Autodesk Fusion 360 part; units mm, degrees
(part 2 of 2)
  dimension "d128" = 3
  constraint coincident A32.centre A41.centre
  constraint coincident A25.centre A40.centre
  constraint coincident A38.centre A43.centre
  constraint coincident A34.centre A42.centre
  measures "d125" diameter of A21
  measures "d126" diameter of A23
  measures "d127" diameter of A24
  measures "d128" diameter of A22
extrude "Extrude11" cut sketch "Sketch4" against normal blind 8 contours A21 | A22 | A23 | A24
extrude "Extrude12" cut sketch "Sketch4" against normal blind 6.5 contours A25 | A32 | A34 | A38 | A40 | A41 | A42 | A43
sketch "Sketch5" plane through (0, 0, 3) normal (0, 0, 1) x (-1, 0, 0)
  circle A0 centre (47, -22) radius 1.5
  circle A1 centre (19.8064, 49.2459) radius 1.5
  circle A2 centre (-21.042, -45.9567) radius 1.5
  circle A3 centre (-47.207, 20.5835) radius 1.5
  circle A4 centre (14, -47) radius 1.5
  circle A5 centre (-47, -14) radius 1.5
  circle A6 centre (47, 14) radius 1.5
  circle A7 centre (-14, 47) radius 1.5
  arc A8 (55, 15) -> (15, 55) centre (15, 15) ccw
  line L0 (15, 55) -> (-15, 55)
  arc A9 (-15, 55) -> (-55, 15) centre (-15, 15) ccw
  line L1 (-55, 15) -> (-55, -15)
  arc A10 (-55, -15) -> (-15, -55) centre (-15, -15) ccw
  line L2 (-15, -55) -> (15, -55)
  arc A11 (15, -55) -> (55, -15) centre (15, -15) ccw
  line L3 (55, -15) -> (55, 15)
  line L4 (41.4394, -9.8393) -> (37.3179, -15.2919)
  spline S0 degree 3 poles (37.3179, -15.2919) (37.6885, -19.157) (38.1371, -22.7222) (37.3203, -26.0559) (37.037, -26.7219) (36.2871, -27.772) (35.8641, -28.165) (34.6133, -28.9678) (33.7328, -29.2635) (32.7908, -29.4916) knots 0 0 0 0 1.164828 1.164828 1.516946 1.516946 1.81941 1.81941 2.270031 2.270031 2.270031 2.270031
  line L5 (32.7908, -29.4916) -> (31.7989, -35.8027)
  line L6 (31.7989, -35.8027) -> (31.0974, -40.2607)
  line L7 (31.0974, -40.2607) -> (33.5883, -40.8482)
  line L8 (33.5883, -40.8482) -> (32.8996, -43.7681)
  line L9 (32.8996, -43.7681) -> (30.6297, -43.2327)
  line L10 (30.6297, -43.2327) -> (29.9635, -47.4663)
  arc A12 (24.1405, -46.0928) -> (29.9635, -47.4663) centre (27, -47) ccw
  line L11 (24.1405, -46.0928) -> (25.4365, -42.0077)
  line L12 (25.4365, -42.0077) -> (23.1667, -41.4723)
  line L13 (23.1667, -41.4723) -> (23.8554, -38.5524)
  line L14 (23.8554, -38.5524) -> (26.3463, -39.14)
  line L15 (26.3463, -39.14) -> (27.7111, -34.8384)
  line L16 (27.7111, -34.8384) -> (28.7703, -30.3481)
  spline S1 degree 3 poles (28.7703, -30.3481) (27.6148, -30.6643) (26.6336, -31.0889) (24.9398, -32.4102) (24.298, -33.1659) (22.092, -36.2546) (20.5653, -39.283) (15.8311, -43.4069) (14.0247, -44.4113) (11.1819, -45.3972) (9.9898, -45.607) (8.1404, -45.5368) (7.3989, -45.3892) (6.1398, -44.8148) (5.64, -44.4531) (4.7208, -43.4815) (4.3496, -42.8831) (3.4629, -41.0501) (3.1013, -39.695) (2.3137, -37.6472) (1.9455, -36.8825) (1.0366, -35.7978) (0.5937, -35.4393) (-0.469, -34.89) (-1.0783, -34.7097) (-3.396, -34.3697) (-5.3987, -34.5812) (-7.6106, -34.9389) knots 0 0 0 0 0.359374 0.359374 0.670478 0.670478 1.446599 1.446599 1.895417 1.895417 2.224922 2.224922 2.450473 2.450473 2.63972 2.63972 2.850158 2.850158 3.247941 3.247941 3.519478 3.519478 3.715617 3.715617 3.915643 3.915643 4.385468 4.385468 4.385468 4.385468
  line L17 (-7.6106, -34.9389) -> (-5.7671, -36.87)
  line L18 (-5.7671, -36.87) -> (-2.4134, -39.8897)
  line L19 (-2.4134, -39.8897) -> (-0.5622, -38.1225)
  line L20 (-0.5622, -38.1225) -> (1.5093, -40.2925)
  line L21 (1.5093, -40.2925) -> (-0.1776, -41.9029)
  line L22 (-0.1776, -41.9029) -> (3.0074, -44.7706)
  arc A13 (-1.3202, -48.9018) -> (3.0074, -44.7706) centre (1, -47) ccw
  line L23 (-1.3202, -48.9018) -> (-4.037, -45.5872)
  line L24 (-4.037, -45.5872) -> (-5.7239, -47.1976)
  line L25 (-5.7239, -47.1976) -> (-7.7954, -45.0276)
  line L26 (-7.7954, -45.0276) -> (-5.9442, -43.2604)
  line L27 (-5.9442, -43.2604) -> (-12.1168, -35.7299)
  spline S2 degree 3 poles (-12.1168, -35.7299) (-14.7803, -36.1844) (-17.4077, -36.5262) (-20.6177, -36.1408) (-21.5954, -35.8949) (-23.1516, -35.0659) (-23.7332, -34.592) (-24.6878, -33.4235) (-25.0394, -32.7732) (-25.5995, -31.3254) (-25.7916, -30.5154) (-25.9192, -29.7135) knots 0 0 0 0 0.810588 0.810588 1.168868 1.168868 1.446193 1.446193 1.71283 1.71283 2.006296 2.006296 2.006296 2.006296
  line L28 (-25.9192, -29.7135) -> (-35.1529, -29.8382)
  line L29 (-35.1529, -29.8382) -> (-39.6653, -29.8999)
  line L30 (-39.6653, -29.8999) -> (-39.8236, -32.4543)
  line L31 (-39.8236, -32.4543) -> (-42.8179, -32.2688)
  line L32 (-42.8179, -32.2688) -> (-42.6736, -29.9411)
  line L33 (-42.6736, -29.9411) -> (-46.959, -29.9997)
  arc A14 (-46.5889, -24.0283) -> (-46.959, -29.9997) centre (-47, -27) ccw
  line L34 (-46.5889, -24.0283) -> (-42.3436, -24.6156)
  line L35 (-42.3436, -24.6156) -> (-42.1994, -22.2879)
  line L36 (-42.1994, -22.2879) -> (-39.2051, -22.4735)
  line L37 (-39.2051, -22.4735) -> (-39.3634, -25.0279)
  line L38 (-39.3634, -25.0279) -> (-34.8931, -25.6463)
  line L39 (-34.8931, -25.6463) -> (-26.1751, -26.1865)
  spline S3 degree 3 poles (-26.1751, -26.1865) (-26.2136, -21.5897) (-25.4228, -16.5889) (-26.5447, -7.6817) (-27.7362, -4.5994) (-31.4465, 2.9635) (-33.9112, 7.1935) (-35.421, 11.5615) knots 0 0 0 0 1.379101 1.379101 2.416171 2.416171 3.558045 3.558045 3.558045 3.558045
  line L40 (-35.421, 11.5615) -> (-38.3057, 7.5335)
  line L41 (-38.3057, 7.5335) -> (-40.6488, 3.6765)
  line L42 (-40.6488, 3.6765) -> (-38.5681, 2.1864)
  line L43 (-38.5681, 2.1864) -> (-40.3148, -0.2527)
  line L44 (-40.3148, -0.2527) -> (-42.2109, 1.1052)
  line L45 (-42.2109, 1.1052) -> (-44.436, -2.5576)
  arc A15 (-49.3002, 0.9259) -> (-44.436, -2.5576) centre (-47, -1) ccw
  line L46 (-49.3002, 0.9259) -> (-46.5489, 4.2119)
  line L47 (-46.5489, 4.2119) -> (-48.445, 5.5698)
  line L48 (-48.445, 5.5698) -> (-46.6982, 8.0088)
  line L49 (-46.6982, 8.0088) -> (-44.6175, 6.5187)
  line L50 (-44.6175, 6.5187) -> (-41.7204, 9.9789)
  line L51 (-41.7204, 9.9789) -> (-36.6853, 17.0096)
  spline S4 degree 3 poles (-36.6853, 17.0096) (-36.8676, 18.8531) (-36.7596, 20.6853) (-35.8249, 23.83) (-35.1927, 25.0859) (-33.4931, 27.4447) (-32.4383, 28.4998) (-31.2814, 29.4234) knots 0 0 0 0 0.555731 0.555731 0.983651 0.983651 1.42815 1.42815 1.42815 1.42815
  line L52 (-31.2814, 29.4234) -> (-30.8456, 35.4405)
  line L53 (-30.8456, 35.4405) -> (-30.5194, 39.9416)
  line L54 (-30.5194, 39.9416) -> (-33.0508, 40.3188)
  line L55 (-33.0508, 40.3188) -> (-32.6086, 43.286)
  line L56 (-32.6086, 43.286) -> (-30.3019, 42.9423)
  line L57 (-30.3019, 42.9423) -> (-29.9922, 47.2169)
  arc A16 (-24.0746, 46.3351) -> (-29.9922, 47.2169) centre (-27, 47) ccw
  line L58 (-24.0746, 46.3351) -> (-25.0245, 42.156)
  line L59 (-25.0245, 42.156) -> (-22.7178, 41.8122)
  line L60 (-22.7178, 41.8122) -> (-23.16, 38.845)
  line L61 (-23.16, 38.845) -> (-25.6913, 39.2222)
  line L62 (-25.6913, 39.2222) -> (-26.6915, 34.8215)
  line L63 (-26.6915, 34.8215) -> (-27.102, 32.0663)
  spline S5 degree 3 poles (-27.102, 32.0663) (-23.8561, 33.7038) (-20.1727, 34.7945) (-13.9908, 35.6095) (-11.9033, 35.3478) (-8.6393, 34.4929) (-7.241, 33.737) (-4.6779, 32.215) (-3.539, 31.4712) (-1.7666, 30.8258) (-1.1355, 30.6903) (0.1203, 30.7222) (0.6844, 30.8607) (1.9595, 31.399) (2.6674, 31.8714) (4.3852, 33.2548) (5.4117, 34.2687) (6.5195, 35.3415) knots 0 0 0 0 1.090679 1.090679 2.116632 2.116632 3.315493 3.315493 4.459674 4.459674 5.071625 5.071625 5.626071 5.626071 6.359803 6.359803 7.369828 7.369828 7.369828 7.369828
  line L64 (6.5195, 35.3415) -> (5.3836, 36.6241)
  line L65 (5.3836, 36.6241) -> (2.1451, 39.7671)
  line L66 (2.1451, 39.7671) -> (0.2292, 38.0703)
  line L67 (0.2292, 38.0703) -> (-1.7598, 40.3162)
  line L68 (-1.7598, 40.3162) -> (-0.0138, 41.8624)
  line L69 (-0.0138, 41.8624) -> (-3.0893, 44.8472)
  arc A17 (1.3897, 48.8137) -> (-3.0893, 44.8472) centre (-1, 47) ccw
  line L70 (1.3897, 48.8137) -> (3.9807, 45.3999)
  line L71 (3.9807, 45.3999) -> (5.7266, 46.946)
  line L72 (5.7266, 46.946) -> (7.7155, 44.7001)
  line L73 (7.7155, 44.7001) -> (5.7996, 43.0034)
  line L74 (5.7996, 43.0034) -> (8.5279, 39.4086)
  line L75 (8.5279, 39.4086) -> (9.6251, 38.1696)
  spline S6 degree 3 poles (9.6251, 38.1696) (11.2124, 39.4725) (12.9202, 40.5975) (16.4323, 41.9003) (18.0613, 42.1653) (21.4266, 42.0265) (23.0731, 41.6295) (26.5653, 40.2029) (28.3145, 39.0547) (30.2985, 37.2379) (30.8783, 36.6163) (31.7822, 35.4004) (32.1434, 34.8061) (32.416, 34.173) knots 0 0 0 0 0.616058 0.616058 1.127035 1.127035 1.633478 1.633478 2.269407 2.269407 2.553154 2.553154 2.787926 2.787926 2.787926 2.787926
  line L76 (32.416, 34.173) -> (36.3135, 32.8488)
  line L77 (36.3135, 32.8488) -> (40.6839, 31.7237)
  line L78 (40.6839, 31.7237) -> (41.5072, 34.147)
  line L79 (41.5072, 34.147) -> (44.3477, 33.1819)
  line L80 (44.3477, 33.1819) -> (43.5975, 30.9737)
  line L81 (43.5975, 30.9737) -> (47.7479, 29.9053)
  arc A18 (45.8232, 24.2404) -> (47.7479, 29.9053) centre (47, 27) ccw
  line L82 (45.8232, 24.2404) -> (41.881, 25.9216)
  line L83 (41.881, 25.9216) -> (41.1307, 23.7134)
  line L84 (41.1307, 23.7134) -> (38.2902, 24.6785)
  line L85 (38.2902, 24.6785) -> (39.1135, 27.1018)
  line L86 (39.1135, 27.1018) -> (34.9623, 28.872)
  line L87 (34.9623, 28.872) -> (33.0026, 29.5379)
  spline S7 degree 3 poles (33.0026, 29.5379) (32.9902, 28.5579) (33.003, 27.1751) (33.5348, 25.6326) (33.7207, 25.3268) (34.1024, 24.8702) (34.3236, 24.7044) (34.8418, 24.4372) (35.1527, 24.347) (36.4443, 24.0711) (37.7665, 23.9707) (40.2586, 22.8614) (41.1591, 22.2488) (42.5804, 20.7638) (43.1055, 19.9446) (43.8206, 18.0888) (43.9818, 17.0988) (44.0027, 14.699) (43.7263, 13.2998) (42.5231, 9.2938) (41.1447, 6.638) (39.093, 2.0196) (38.3333, 0.1029) (37.2326, -4.3021) (36.9907, -6.4921) (36.9644, -8.7943) knots 0 0 0 0 0.294006 0.294006 0.417435 0.417435 0.550082 0.550082 0.704478 0.704478 1.129194 1.129194 1.408869 1.408869 1.66214 1.66214 1.922723 1.922723 2.2812 2.2812 3.001747 3.001747 3.492602 3.492602 4.002499 4.002499 4.002499 4.002499
  line L88 (36.9644, -8.7943) -> (38.0888, -7.3067)
  line L89 (38.0888, -7.3067) -> (40.5305, -3.5114)
  line L90 (40.5305, -3.5114) -> (38.4888, -1.9682)
  line L91 (38.4888, -1.9682) -> (40.2978, 0.4251)
  line L92 (40.2978, 0.4251) -> (42.1583, -0.9812)
  line L93 (42.1583, -0.9812) -> (44.477, 2.6231)
  arc A19 (49.2498, -0.9845) -> (44.477, 2.6231) centre (47, 1) ccw
  line L94 (49.2498, -0.9845) -> (46.4148, -4.1986)
  line L95 (46.4148, -4.1986) -> (48.2753, -5.6048)
  line L96 (48.2753, -5.6048) -> (46.4663, -7.9981)
  line L97 (46.4663, -7.9981) -> (44.4246, -6.4548)
  line L98 (44.4246, -6.4548) -> (41.4394, -9.8393)
  circle A20 centre (37.75, -38.15) radius 2.75
  circle A21 centre (38.15, 37.75) radius 2.75
  circle A22 centre (-38.15, -37.75) radius 2.75
  circle A23 centre (-37.75, 38.15) radius 2.75
  circle A24 centre (19.8064, 49.2459) radius 4
  line L99 (23.8064, 49.2459) -> (23.8064, 54.0186)
  line L100 (15.8064, 49.2459) -> (15.8064, 54.9919)
  dimension "d133" = 8
  constraint concentric A1 A24
  constraint coincident A24 L99.start
  constraint coincident A8 L99.end
  constraint tangent A24 L99
  constraint vertical L99
  constraint coincident A24 L100.start
  constraint coincident A8 L100.end
  constraint tangent A24 L100
  constraint vertical L100
  measures "d133" diameter of A24
sketch "LaserMidPlateShellBearing" plane through (0, 0, 3) normal (0, 0, 1) x (-1, 0, 0)
  circle A0 centre (47, -22) radius 1.5
  circle A1 centre (19.8064, 49.2459) radius 1.5
  circle A2 centre (-21.042, -45.9567) radius 1.5
  circle A3 centre (-47.207, 20.5835) radius 1.5
  circle A4 centre (14, -47) radius 1.5
  circle A5 centre (-47, -14) radius 1.5
  circle A6 centre (47, 14) radius 1.5
  circle A7 centre (-14, 47) radius 1.5
  arc A8 (55, 15) -> (15, 55) centre (15, 15) ccw
  line L0 (15, 55) -> (-15, 55)
  arc A9 (-15, 55) -> (-55, 15) centre (-15, 15) ccw
  line L1 (-55, 15) -> (-55, -15)
  arc A10 (-55, -15) -> (-15, -55) centre (-15, -15) ccw
  line L2 (-15, -55) -> (15, -55)
  arc A11 (15, -55) -> (55, -15) centre (15, -15) ccw
  line L3 (55, -15) -> (55, 15)
  line L4 (41.4394, -9.8393) -> (37.3179, -15.2919)
  spline S0 degree 3 poles (37.3179, -15.2919) (37.6885, -19.157) (38.1371, -22.7222) (37.3203, -26.0559) (37.037, -26.7219) (36.2871, -27.772) (35.8641, -28.165) (34.6133, -28.9678) (33.7328, -29.2635) (32.7908, -29.4916) knots 0 0 0 0 1.164828 1.164828 1.516946 1.516946 1.81941 1.81941 2.270031 2.270031 2.270031 2.270031
  line L5 (32.7908, -29.4916) -> (31.7989, -35.8027)
  line L6 (31.7989, -35.8027) -> (31.0974, -40.2607)
  line L7 (31.0974, -40.2607) -> (33.5883, -40.8482)
  line L8 (33.5883, -40.8482) -> (32.8996, -43.7681)
  line L9 (32.8996, -43.7681) -> (30.6297, -43.2327)
  line L10 (30.6297, -43.2327) -> (29.9635, -47.4663)
  arc A12 (24.1405, -46.0928) -> (29.9635, -47.4663) centre (27, -47) ccw
  line L11 (24.1405, -46.0928) -> (25.4365, -42.0077)
  line L12 (25.4365, -42.0077) -> (23.1667, -41.4723)
  line L13 (23.1667, -41.4723) -> (23.8554, -38.5524)
  line L14 (23.8554, -38.5524) -> (26.3463, -39.14)
  line L15 (26.3463, -39.14) -> (27.7111, -34.8384)
  line L16 (27.7111, -34.8384) -> (28.7703, -30.3481)
  spline S1 degree 3 poles (28.7703, -30.3481) (27.6148, -30.6643) (26.6336, -31.0889) (24.9398, -32.4102) (24.298, -33.1659) (22.092, -36.2546) (20.5653, -39.283) (15.8311, -43.4069) (14.0247, -44.4113) (11.1819, -45.3972) (9.9898, -45.607) (8.1404, -45.5368) (7.3989, -45.3892) (6.1398, -44.8148) (5.64, -44.4531) (4.7208, -43.4815) (4.3496, -42.8831) (3.4629, -41.0501) (3.1013, -39.695) (2.3137, -37.6472) (1.9455, -36.8825) (1.0366, -35.7978) (0.5937, -35.4393) (-0.469, -34.89) (-1.0783, -34.7097) (-3.396, -34.3697) (-5.3987, -34.5812) (-7.6106, -34.9389) knots 0 0 0 0 0.359374 0.359374 0.670478 0.670478 1.446599 1.446599 1.895417 1.895417 2.224922 2.224922 2.450473 2.450473 2.63972 2.63972 2.850158 2.850158 3.247941 3.247941 3.519478 3.519478 3.715617 3.715617 3.915643 3.915643 4.385468 4.385468 4.385468 4.385468
  line L17 (-7.6106, -34.9389) -> (-5.7671, -36.87)
  line L18 (-5.7671, -36.87) -> (-2.4134, -39.8897)
  line L19 (-2.4134, -39.8897) -> (-0.5622, -38.1225)
  line L20 (-0.5622, -38.1225) -> (1.5093, -40.2925)
  line L21 (1.5093, -40.2925) -> (-0.1776, -41.9029)
  line L22 (-0.1776, -41.9029) -> (3.0074, -44.7706)
  arc A13 (-1.3202, -48.9018) -> (3.0074, -44.7706) centre (1, -47) ccw
  line L23 (-1.3202, -48.9018) -> (-4.037, -45.5872)
  line L24 (-4.037, -45.5872) -> (-5.7239, -47.1976)
  line L25 (-5.7239, -47.1976) -> (-7.7954, -45.0276)
  line L26 (-7.7954, -45.0276) -> (-5.9442, -43.2604)
  line L27 (-5.9442, -43.2604) -> (-12.1168, -35.7299)
  spline S2 degree 3 poles (-12.1168, -35.7299) (-14.7803, -36.1844) (-17.4077, -36.5262) (-20.6177, -36.1408) (-21.5954, -35.8949) (-23.1516, -35.0659) (-23.7332, -34.592) (-24.6878, -33.4235) (-25.0394, -32.7732) (-25.5995, -31.3254) (-25.7916, -30.5154) (-25.9192, -29.7135) knots 0 0 0 0 0.810588 0.810588 1.168868 1.168868 1.446193 1.446193 1.71283 1.71283 2.006296 2.006296 2.006296 2.006296
  line L28 (-25.9192, -29.7135) -> (-35.1529, -29.8382)
  line L29 (-35.1529, -29.8382) -> (-39.6653, -29.8999)
  line L30 (-39.6653, -29.8999) -> (-39.8236, -32.4543)
  line L31 (-39.8236, -32.4543) -> (-42.8179, -32.2688)
  line L32 (-42.8179, -32.2688) -> (-42.6736, -29.9411)
  line L33 (-42.6736, -29.9411) -> (-46.959, -29.9997)
  arc A14 (-46.5889, -24.0283) -> (-46.959, -29.9997) centre (-47, -27) ccw
  line L34 (-46.5889, -24.0283) -> (-42.3436, -24.6156)
  line L35 (-42.3436, -24.6156) -> (-42.1994, -22.2879)
  line L36 (-42.1994, -22.2879) -> (-39.2051, -22.4735)
  line L37 (-39.2051, -22.4735) -> (-39.3634, -25.0279)
  line L38 (-39.3634, -25.0279) -> (-34.8931, -25.6463)
  line L39 (-34.8931, -25.6463) -> (-26.1751, -26.1865)
  spline S3 degree 3 poles (-26.1751, -26.1865) (-26.2136, -21.5897) (-25.4228, -16.5889) (-26.5447, -7.6817) (-27.7362, -4.5994) (-31.4465, 2.9635) (-33.9112, 7.1935) (-35.421, 11.5615) knots 0 0 0 0 1.379101 1.379101 2.416171 2.416171 3.558045 3.558045 3.558045 3.558045
  line L40 (-35.421, 11.5615) -> (-38.3057, 7.5335)
  line L41 (-38.3057, 7.5335) -> (-40.6488, 3.6765)
  line L42 (-40.6488, 3.6765) -> (-38.5681, 2.1864)
  line L43 (-38.5681, 2.1864) -> (-40.3148, -0.2527)
  line L44 (-40.3148, -0.2527) -> (-42.2109, 1.1052)
  line L45 (-42.2109, 1.1052) -> (-44.436, -2.5576)
  arc A15 (-49.3002, 0.9259) -> (-44.436, -2.5576) centre (-47, -1) ccw
  line L46 (-49.3002, 0.9259) -> (-46.5489, 4.2119)
  line L47 (-46.5489, 4.2119) -> (-48.445, 5.5698)
  line L48 (-48.445, 5.5698) -> (-46.6982, 8.0088)
  line L49 (-46.6982, 8.0088) -> (-44.6175, 6.5187)
  line L50 (-44.6175, 6.5187) -> (-41.7204, 9.9789)
  line L51 (-41.7204, 9.9789) -> (-36.6853, 17.0096)
  spline S4 degree 3 poles (-36.6853, 17.0096) (-36.8676, 18.8531) (-36.7596, 20.6853) (-35.8249, 23.83) (-35.1927, 25.0859) (-33.4931, 27.4447) (-32.4383, 28.4998) (-31.2814, 29.4234) knots 0 0 0 0 0.555731 0.555731 0.983651 0.983651 1.42815 1.42815 1.42815 1.42815
  line L52 (-31.2814, 29.4234) -> (-30.8456, 35.4405)
  line L53 (-30.8456, 35.4405) -> (-30.5194, 39.9416)
  line L54 (-30.5194, 39.9416) -> (-33.0508, 40.3188)
  line L55 (-33.0508, 40.3188) -> (-32.6086, 43.286)
  line L56 (-32.6086, 43.286) -> (-30.3019, 42.9423)
  line L57 (-30.3019, 42.9423) -> (-29.9922, 47.2169)
  arc A16 (-24.0746, 46.3351) -> (-29.9922, 47.2169) centre (-27, 47) ccw
  line L58 (-24.0746, 46.3351) -> (-25.0245, 42.156)
  line L59 (-25.0245, 42.156) -> (-22.7178, 41.8122)
  line L60 (-22.7178, 41.8122) -> (-23.16, 38.845)
  line L61 (-23.16, 38.845) -> (-25.6913, 39.2222)
  line L62 (-25.6913, 39.2222) -> (-26.6915, 34.8215)
  line L63 (-26.6915, 34.8215) -> (-27.102, 32.0663)
  spline S5 degree 3 poles (-27.102, 32.0663) (-23.8561, 33.7038) (-20.1727, 34.7945) (-13.9908, 35.6095) (-11.9033, 35.3478) (-8.6393, 34.4929) (-7.241, 33.737) (-4.6779, 32.215) (-3.539, 31.4712) (-1.7666, 30.8258) (-1.1355, 30.6903) (0.1203, 30.7222) (0.6844, 30.8607) (1.9595, 31.399) (2.6674, 31.8714) (4.3852, 33.2548) (5.4117, 34.2687) (6.5195, 35.3415) knots 0 0 0 0 1.090679 1.090679 2.116632 2.116632 3.315493 3.315493 4.459674 4.459674 5.071625 5.071625 5.626071 5.626071 6.359803 6.359803 7.369828 7.369828 7.369828 7.369828
  line L64 (6.5195, 35.3415) -> (5.3836, 36.6241)
  line L65 (5.3836, 36.6241) -> (2.1451, 39.7671)
  line L66 (2.1451, 39.7671) -> (0.2292, 38.0703)
  line L67 (0.2292, 38.0703) -> (-1.7598, 40.3162)
  line L68 (-1.7598, 40.3162) -> (-0.0138, 41.8624)
  line L69 (-0.0138, 41.8624) -> (-3.0893, 44.8472)
  arc A17 (1.3897, 48.8137) -> (-3.0893, 44.8472) centre (-1, 47) ccw
  line L70 (1.3897, 48.8137) -> (3.9807, 45.3999)
  line L71 (3.9807, 45.3999) -> (5.7266, 46.946)
  line L72 (5.7266, 46.946) -> (7.7155, 44.7001)
  line L73 (7.7155, 44.7001) -> (5.7996, 43.0034)
  line L74 (5.7996, 43.0034) -> (8.5279, 39.4086)
  line L75 (8.5279, 39.4086) -> (9.6251, 38.1696)
  spline S6 degree 3 poles (9.6251, 38.1696) (11.2124, 39.4725) (12.9202, 40.5975) (16.4323, 41.9003) (18.0613, 42.1653) (21.4266, 42.0265) (23.0731, 41.6295) (26.5653, 40.2029) (28.3145, 39.0547) (30.2985, 37.2379) (30.8783, 36.6163) (31.7822, 35.4004) (32.1434, 34.8061) (32.416, 34.173) knots 0 0 0 0 0.616058 0.616058 1.127035 1.127035 1.633478 1.633478 2.269407 2.269407 2.553154 2.553154 2.787926 2.787926 2.787926 2.787926
  line L76 (32.416, 34.173) -> (36.3135, 32.8488)
  line L77 (36.3135, 32.8488) -> (40.6839, 31.7237)
  line L78 (40.6839, 31.7237) -> (41.5072, 34.147)
  line L79 (41.5072, 34.147) -> (44.3477, 33.1819)
  line L80 (44.3477, 33.1819) -> (43.5975, 30.9737)
  line L81 (43.5975, 30.9737) -> (47.7479, 29.9053)
  arc A18 (45.8232, 24.2404) -> (47.7479, 29.9053) centre (47, 27) ccw
  line L82 (45.8232, 24.2404) -> (41.881, 25.9216)
  line L83 (41.881, 25.9216) -> (41.1307, 23.7134)
  line L84 (41.1307, 23.7134) -> (38.2902, 24.6785)
  line L85 (38.2902, 24.6785) -> (39.1135, 27.1018)
  line L86 (39.1135, 27.1018) -> (34.9623, 28.872)
  line L87 (34.9623, 28.872) -> (33.0026, 29.5379)
  spline S7 degree 3 poles (33.0026, 29.5379) (32.9902, 28.5579) (33.003, 27.1751) (33.5348, 25.6326) (33.7207, 25.3268) (34.1024, 24.8702) (34.3236, 24.7044) (34.8418, 24.4372) (35.1527, 24.347) (36.4443, 24.0711) (37.7665, 23.9707) (40.2586, 22.8614) (41.1591, 22.2488) (42.5804, 20.7638) (43.1055, 19.9446) (43.8206, 18.0888) (43.9818, 17.0988) (44.0027, 14.699) (43.7263, 13.2998) (42.5231, 9.2938) (41.1447, 6.638) (39.093, 2.0196) (38.3333, 0.1029) (37.2326, -4.3021) (36.9907, -6.4921) (36.9644, -8.7943) knots 0 0 0 0 0.294006 0.294006 0.417435 0.417435 0.550082 0.550082 0.704478 0.704478 1.129194 1.129194 1.408869 1.408869 1.66214 1.66214 1.922723 1.922723 2.2812 2.2812 3.001747 3.001747 3.492602 3.492602 4.002499 4.002499 4.002499 4.002499
  line L88 (36.9644, -8.7943) -> (38.0888, -7.3067)
  line L89 (38.0888, -7.3067) -> (40.5305, -3.5114)
  line L90 (40.5305, -3.5114) -> (38.4888, -1.9682)
  line L91 (38.4888, -1.9682) -> (40.2978, 0.4251)
  line L92 (40.2978, 0.4251) -> (42.1583, -0.9812)
  line L93 (42.1583, -0.9812) -> (44.477, 2.6231)
  arc A19 (49.2498, -0.9845) -> (44.477, 2.6231) centre (47, 1) ccw
  line L94 (49.2498, -0.9845) -> (46.4148, -4.1986)
  line L95 (46.4148, -4.1986) -> (48.2753, -5.6048)
  line L96 (48.2753, -5.6048) -> (46.4663, -7.9981)
  line L97 (46.4663, -7.9981) -> (44.4246, -6.4548)
  line L98 (44.4246, -6.4548) -> (41.4394, -9.8393)
  circle A20 centre (37.75, -38.15) radius 2.75
  circle A21 centre (38.15, 37.75) radius 2.75
  circle A22 centre (-38.15, -37.75) radius 2.75
  circle A23 centre (-37.75, 38.15) radius 2.75
